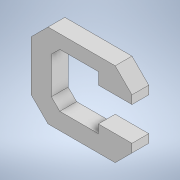
# Autodesk Inventor part: Assignment 2.1 - C-Clip
Saved by Autodesk Inventor 2021.1 (Build 251245000, 245)
## iProperties
Created: 2021-05-13
Part Number: Assignment 2.1 - C-Clip
Material: Generic
Document SubType Name: Modeling
Designer: as000166
Density: 1 g/cm^3
Appearance: Default
Author: as000166
Autodesk Inventor part; units mm, degrees
ref_plane "YZ Plane" through (0, 0, 0) normal (1, 0, 0) x (0, 1, 0)
ref_plane "XZ Plane" through (0, 0, 0) normal (0, 1, 0) x (-1, 0, 0)
ref_plane "XY Plane" through (0, 0, 0) normal (0, 0, 1) x (1, 0, 0)
sketch "Sketch1" plane through (0, 0, 0) normal (0, 0, 1) x (1, 0, 0)
  line L0 (0, 0) -> (25.4, 0)
  line L1 (-6.35, 6.35) -> (0, 0)
  line L2 (31.75, 6.35) -> (25.4, 0)
  line L3 (-6.35, 6.35) -> (-6.35, 25.4)
  line L4 (-6.35, 25.4) -> (0, 31.75)
  line L5 (0, 31.75) -> (25.4, 31.75)
  line L6 (25.4, 31.75) -> (31.75, 25.4)
  line L7 (31.75, 25.4) -> (31.75, 22.225)
  line L8 (31.75, 22.225) -> (19.05, 22.225)
  line L9 (19.05, 26.67) -> (19.05, 22.225)
  line L10 (1.27, 19.05) -> (1.27, 9.525)
  line L11 (4.445, 6.35) -> (1.27, 9.525)
  line L12 (1.27, 19.05) -> (1.27, 23.495)
  line L13 (4.445, 26.67) -> (1.27, 23.495)
  line L14 (31.75, 6.35) -> (31.75, 9.525)
  line L15 (31.75, 9.525) -> (19.05, 9.525)
  line L16 (19.05, 9.525) -> (19.05, 6.35)
  line L17 (19.05, 6.35) -> (4.445, 6.35)
  line L18 (4.445, 26.67) -> (19.05, 26.67)
  dimension "d0" = 25.4
  dimension "d6" = 19.05
  dimension "d7" = 25.4
  dimension "d8" = 3.175
  dimension "d9" = 12.7
  dimension "d21" = 3.175
  dimension "d22" = 12.7
  dimension "d23" = 3.175
  constraints: 38 end point, 7 perpendicular, 4 vertical, 1 horizontal, 1 parallel
  measures "d0" distance of L0.start L0.end
  measures "d6" distance of L1.start L3.end
  measures "d7" distance of L4.end L5.end
  measures "d8" distance of L6.end L7.end
  measures "d9" distance of L7.end L8.end
  measures "d21" distance of L2.start L14.end
  measures "d22" distance of L14.end L15.end
  measures "d23" distance of L15.end L16.end
extrude "Extrusion1" add sketch "Sketch1" along normal blind 6.35
body "Solid1"
